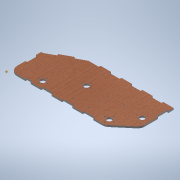
# Autodesk Inventor part: Frame wiel binnen
Saved by Autodesk Inventor 2021 (Build 250183000, 183)
## iProperties
Manager: PJ / DCS
Company: Emmaüs Bovenbouw Aalter
Created: 2020-10-22
Part Number: Frame wiel binnen
Material: S235
Catalog Web Link: http://emmausbovenbouw.op-weg.be/
Vendor: Emmaüsinstituut Bovenbouw Aalter
Document SubType Name: Modeling
Designer: Antho
Engineer: Declercq St.
Manufacturer: Standard
Standards Organization: Custom
Density: 7.86 g/cm^3
Appearance: Steel
Title: Algemene titel
Subject: Specifieke titel
Author: Antho
Keywords: Ruwe Ø xxxxx
Comments: Opmerking
Autodesk Inventor part; units mm, degrees
ref_plane "YZ Plane" through (0, 0, 0) normal (1, 0, 0) x (0, 1, 0)
ref_plane "XZ Plane" through (0, 0, 0) normal (0, 1, 0) x (-1, 0, 0)
ref_plane "XY Plane" through (0, 0, 0) normal (0, 0, 1) x (1, 0, 0)
sketch "Sketch7" plane through (0, 0, 0) normal (0, 0, 1) x (1, 0, 0)
  line L0 (0, 0) -> (0, 51)
  line L1 (340, 102) -> (340, 51)
  line L2 (280, 0) -> (0, 0)
  line L3 (0, 0) -> (0, 30)
  line L4 (280, 0) -> (340, 51)
  line L5 (0, 51) -> (0, 151)
  line L6 (0, 151) -> (340, 151)
  line L7 (340, 102) -> (340, 151)
  line L8 (335, 146) -> (335, 102)
  line L9 (335, 102) -> (335, 53.3122)
  line L10 (335, 53.3122) -> (278.1621, 5)
  line L11 (278.1621, 5) -> (5, 5)
  line L12 (5, 5) -> (5, 51)
  line L13 (5, 51) -> (5, 146)
  line L14 (5, 146) -> (335, 146)
  dimension "d56" = 51
  dimension "d60" = 51
  dimension "d79" = 100
  dimension "d81" = 5
  constraints: 30 end point, 4 perpendicular, 2 vertical, 1 point on line, 6 other
  measures "d56" distance of L0.start L0.end
  measures "d60" distance of L1.start L1.end
  measures "d79" distance of L0.end L5.end
  measures "d81" distance between parallel lines of L6 L14
extrude "Extrusion3" add sketch "Sketch7" along normal blind 5 contours L0 L5 L6 L7 L1 L4 L2 | L8 L9 L10 L11 L12 L13 L14
fillet "Fillet1" radius 25.5 3 edges at (280, 0, 2.5) (340, 51, 2.5) (0, 0, 2.5)
sketch "Sketch9" plane through (0, 0, 5) normal (0, 0, 1) x (1, 0, 0)
  arc A0 (0, 25.5) -> (25.5, 0) centre (25.5, 25.5) ccw projected
  arc A1 (270.6268, 0) -> (287.1418, 6.0705) centre (270.6268, 25.5) ccw projected
  arc A2 (340, 76.5) -> (314.5, 102) centre (314.5, 76.5) ccw projected
  arc A3 (154.2165, 102) -> (146.008, 100.6427) centre (154.2165, 76.5) ccw projected
  point P0 (0, 0)
  constraints: 3 coincident
hole "Hole4" at (154.2165, 76.5, 5) at (314.5, 76.5, 5) at (270.6268, 25.5, 5) direction (0, 0, -1) diameter 15 end through all
sketch "Sketch13" plane through (0, 0, 5) normal (0, 0, 1) x (1, 0, 0)
  circle A0 centre (154.2165, 76.5) radius 7.5 projected
  line L0 (25.5, 25.5) -> (154.2165, 76.5)
  line L1 (154.2165, 76.5) -> (100.2948, 55.1352)
  line L2 (25.5, 25.5) -> (79.4217, 46.8648)
  line L3 (25.5, 25.5) -> (83.5, 25.5)
  line L4 (154.2165, 76.5) -> (154.2165, 18.5)
  circle A1 centre (270.6268, 25.5) radius 7.5 projected
  line L5 (270.6268, 25.5) -> (212.6268, 25.5)
  circle A2 centre (270.6268, 25.5) radius 58
  circle A3 centre (314.5, 76.5) radius 7.5 projected
  circle A4 centre (314.5, 76.5) radius 58
  line L6 (256.7439, 81.814) -> (177.9806, 81.814)
  line L7 (154.2165, 76.5) -> (211.9725, 81.814)
  point P0 (0, 0)
  dimension "d89" = 116
  dimension "d90" = 116
  dimension "d84" = 58
  dimension "d85" = 58
  dimension "d86" = 58
  dimension "d87" = 58
  dimension "d88" = 58
  dimension "d91" = 58
  constraints: 16 end point, 5 coincident, 3 horizontal, 3 point on line, 1 vertical, 6 other
  measures "d84" distance of L0.end L1.end
  measures "d85" distance of L0.start L2.end
  measures "d86" distance of L0.start L3.end
  measures "d87" distance of L0.end L4.end
  measures "d88" distance of L5.start L5.end
  measures "d91" distance of L0.end L7.end
hole "Hole5" at (212.6268, 25.5, 5) at (211.9725, 81.814, 5) at (256.7439, 81.814, 5) direction (0, 0, -1) diameter 4 depth 8
thicken "Thicken1" operation add thickness 5 both sides no extend neighbours yes toward (0, 1, 0) faces at (107.2089, 0, 1.6667) (6.8072, 8.1556, 1.6667) (272.6208, 0.0781, 1.6667) (301.7662, 18.5013, 1.6667) (338.3567, 53.7863, 1.6667) (340, 92.1948, 1.6667) (226.6667, 151, 1.6667) (0, 109.1667, 1.6667)
sketch "Sketch14" plane through (0, 0, 5) normal (0, 0, 1) x (1, 0, 0)
  line L0 (5, 146) -> (5, 25.5) projected
  line L1 (5, 25.5) -> (5, 5)
  line L2 (25.5, 5) -> (270.6268, 5) projected
  line L3 (5, 5) -> (35, 5)
  line L4 (35, 5) -> (65, 5)
  line L5 (65, 5) -> (95, 5)
  line L6 (95, 5) -> (125, 5)
  line L7 (125, 5) -> (155, 5)
  line L8 (155, 5) -> (185, 5)
  line L9 (185, 5) -> (215, 5)
  line L10 (215, 5) -> (245, 5)
  line L11 (245, 5) -> (275, 5)
  line L12 (35, 5) -> (65, 5)
  line L13 (65, 5) -> (65, 10)
  line L14 (65, 10) -> (50, 10)
  line L15 (35, 13) -> (35, 5)
  line L16 (95, 5) -> (125, 5)
  line L17 (125, 5) -> (125, 10)
  line L18 (125, 10) -> (95, 10)
  line L19 (95, 10) -> (95, 5)
  line L20 (155, 5) -> (185, 5)
  line L21 (185, 5) -> (185, 10)
  line L22 (185, 10) -> (155, 10)
  line L23 (155, 10) -> (155, 5)
  line L24 (215, 5) -> (245, 5)
  line L25 (245, 5) -> (245, 10)
  line L26 (245, 10) -> (215, 10)
  line L27 (215, 10) -> (215, 5)
  line L28 (65, 5) -> (50, 5)
  line L29 (50, 5) -> (50, 10)
  line L30 (50, 10) -> (65, 10)
  line L31 (65, 10) -> (65, 5)
  point P0 (0, 0)
  dimension "d102" = 30
  dimension "d103" = 30
  dimension "d104" = 30
  dimension "d105" = 30
  dimension "d106" = 30
  dimension "d107" = 30
  dimension "d109" = 30
  dimension "d110" = 30
  dimension "d111" = 30
  dimension "d113" = 5
  dimension "d114" = 30
  dimension "d115" = 30
  dimension "d118" = 15
  constraints: 60 end point, 12 point on line, 10 parallel, 6 perpendicular, 5 horizontal
  measures "d102" distance of L1.end L3.end
  measures "d103" distance of L3.end L4.end
  measures "d104" distance of L4.end L5.end
  measures "d105" distance of L5.end L6.end
  measures "d106" distance of L6.end L7.end
  measures "d107" distance of L7.end L8.end
  measures "d109" distance of L8.end L9.end
  measures "d110" distance of L9.end L10.end
  measures "d111" distance of L10.end L11.end
  measures "d113" distance of L13.end L12.end
  measures "d114" distance of L18.end L17.end
  measures "d115" distance of L22.end L21.end
  measures "d118" distance of L14.end L30.end
extrude "Extrusion4" cut sketch "Sketch14" against normal blind 10
sketch "Sketch15" plane through (0, 0, 5) normal (0, 0, 1) x (1, 0, 0)
  line L0 (25.5, 5) -> (50, 5) projected
  line L1 (25.5, 5) -> (5, 5)
  arc A0 (5, 25.5) -> (25.5, 5) centre (25.5, 25.5) ccw projected
  line L2 (5, 5) -> (5, 50)
  line L3 (5, 146) -> (5, 25.5) projected
  line L4 (5, 50) -> (5, 80)
  line L5 (5, 80) -> (5, 110)
  line L6 (5, 110) -> (5, 80)
  line L7 (5, 80) -> (5, 110)
  line L8 (5, 110) -> (5, 138)
  line L9 (5, 50) -> (10, 50)
  line L10 (10, 50) -> (10, 80)
  line L11 (10, 80) -> (5, 80)
  line L12 (5, 80) -> (5, 50)
  line L13 (5, 110) -> (10, 110)
  line L14 (10, 110) -> (10, 146)
  line L15 (10, 146) -> (5, 146)
  line L16 (5, 146) -> (5, 110)
  line L17 (5, 110) -> (10, 110)
  line L18 (10, 110) -> (10, 138)
  line L19 (10, 138) -> (5, 138)
  line L20 (5, 138) -> (5, 110)
  point P0 (0, 0)
  point P1 (5, 138)
  dimension "d119" = 45
  dimension "d120" = 30
  dimension "d121" = 30
  dimension "d122" = 30
  dimension "d123" = 30
  dimension "d124" = 28
  dimension "d125" = 5
  dimension "d148" = 28
  constraints: 38 end point, 6 parallel, 6 point on line, 4 horizontal, 3 perpendicular, 2 collinear, 1 tangent
  measures "d119" distance of L1.end L2.end
  measures "d120" distance of L2.end L4.end
  measures "d121" distance of L4.end L5.end
  measures "d122" distance of L5.end L4.end
  measures "d123" distance of L4.end L5.end
  measures "d124" distance of L5.end L8.end
  measures "d125" distance of L11.end L10.end
  measures "d148" distance of L17.end L18.end
extrude "Extrusion5" cut sketch "Sketch15" against normal blind 10 contours L19 L14 L13 L3 | L11 L10 L9 L3
sketch "Sketch16" plane through (0, 0, 5) normal (0, 0, 1) x (1, 0, 0)
  line L0 (335, 146) -> (5, 146) projected
  line L1 (5, 146) -> (35, 146)
  line L2 (35, 146) -> (65, 146)
  line L3 (65, 146) -> (95, 146)
  line L4 (95, 146) -> (125, 146)
  line L5 (125, 146) -> (155, 146)
  line L6 (155, 146) -> (185, 146)
  line L7 (185, 146) -> (215, 146)
  line L8 (215, 146) -> (245, 146)
  line L9 (245, 146) -> (275, 146)
  line L10 (275, 146) -> (305, 146)
  line L11 (305, 146) -> (335, 146)
  line L12 (5, 146) -> (35, 146)
  line L13 (35, 146) -> (35, 141)
  line L14 (35, 141) -> (5, 141)
  line L15 (5, 141) -> (5, 146)
  line L16 (65, 146) -> (95, 146)
  line L17 (95, 146) -> (95, 141)
  line L18 (95, 141) -> (65, 141)
  line L19 (65, 141) -> (65, 146)
  line L20 (125, 146) -> (155, 146)
  line L21 (155, 146) -> (155, 141)
  line L22 (155, 141) -> (125, 141)
  line L23 (125, 141) -> (125, 146)
  line L24 (185, 146) -> (215, 146)
  line L25 (215, 146) -> (215, 141)
  line L26 (215, 141) -> (185, 141)
  line L27 (185, 141) -> (185, 146)
  line L28 (245, 146) -> (275, 146)
  line L29 (275, 146) -> (275, 141)
  line L30 (275, 141) -> (245, 141)
  line L31 (245, 141) -> (245, 146)
  line L32 (335, 62.7922) -> (335, 146) projected
  line L33 (305, 146) -> (335, 146)
  line L34 (335, 146) -> (335, 141)
  line L35 (335, 141) -> (305, 141)
  line L36 (305, 141) -> (305, 146)
  line L37 (35, 146) -> (65, 146)
  line L38 (65, 146) -> (65, 141)
  line L39 (65, 141) -> (35, 141)
  line L40 (35, 141) -> (35, 146)
  line L41 (95, 146) -> (125, 146)
  line L42 (125, 146) -> (125, 141)
  line L43 (125, 141) -> (95, 141)
  line L44 (95, 141) -> (95, 146)
  line L45 (155, 146) -> (185, 146)
  line L46 (185, 146) -> (185, 141)
  line L47 (185, 141) -> (155, 141)
  line L48 (155, 141) -> (155, 146)
  line L49 (215, 146) -> (245, 146)
  line L50 (245, 146) -> (245, 141)
  line L51 (245, 141) -> (215, 141)
  line L52 (215, 141) -> (215, 146)
  line L53 (275, 146) -> (305, 146)
  line L54 (305, 146) -> (305, 141)
  line L55 (305, 141) -> (275, 141)
  line L56 (275, 141) -> (275, 146)
  point P0 (0, 0)
  dimension "d128" = 30
  dimension "d129" = 30
  dimension "d130" = 30
  dimension "d131" = 30
  dimension "d132" = 30
  dimension "d133" = 30
  dimension "d134" = 30
  dimension "d135" = 30
  dimension "d136" = 30
  dimension "d137" = 30
  dimension "d138" = 30
  dimension "d139" = 5
  constraints: 110 end point, 23 equal length, 11 horizontal, 11 perpendicular, 6 point on line, 11 other
  measures "d128" distance of L1.start L1.end
  measures "d129" distance of L1.end L2.end
  measures "d130" distance of L2.end L3.end
  measures "d131" distance of L3.end L4.end
  measures "d132" distance of L4.end L5.end
  measures "d133" distance of L5.end L6.end
  measures "d134" distance of L6.end L7.end
  measures "d135" distance of L7.end L8.end
  measures "d136" distance of L8.end L9.end
  measures "d137" distance of L9.end L10.end
  measures "d138" distance of L10.end L11.end
  measures "d139" distance of L12.end L13.end
extrude "Extrusion6" cut sketch "Sketch16" against normal blind 10 contours L36 L55 L29 L0 | L31 L51 L25 L0 | L27 L47 L21 L0 | L23 L43 L17 L0 | L19 L39 L13 L0
sketch "Sketch17" plane through (0, 0, 5) normal (0, 0, 1) x (1, 0, 0)
  line L0 (335, 146) -> (305, 146) projected
  line L1 (335, 146) -> (335, 131)
  line L2 (335, 62.7922) -> (335, 146) projected
  line L3 (335, 131) -> (335, 101)
  line L4 (335, 101) -> (335, 71)
  line L5 (335, 101) -> (330, 101)
  line L6 (330, 101) -> (330, 131)
  line L7 (330, 131) -> (335, 131)
  line L8 (335, 131) -> (335, 101)
  point P0 (0, 0)
  dimension "d142" = 15
  dimension "d143" = 30
  dimension "d144" = 30
  dimension "d145" = 5
  constraints: 14 end point, 3 point on line, 2 parallel, 1 horizontal, 1 perpendicular
  measures "d142" distance of L0.start L1.end
  measures "d143" distance of L1.end L3.end
  measures "d144" distance of L3.end L4.end
  measures "d145" distance of L6.end L7.end
extrude "Extrusion7" cut sketch "Sketch17" against normal blind 10
sketch "Sketch18" plane through (0, 0, 5) normal (0, 0, 1) x (1, 0, 0)
  circle A0 centre (314.5, 76.5) radius 7.5 projected
  circle A1 centre (314.5, 76.5) radius 16
  line L0 (314.5, 76.5) -> (314.5, 60.5)
  line L1 (314.5, 76.5) -> (298.5, 76.5)
  line L2 (314.5, 76.5) -> (314.5, 92.5)
  point P0 (0, 0)
  dimension "d149" = 32
  constraints: 6 end point, 4 coincident, 3 point on circle, 1 centre point, 1 perpendicular, 1 point on line, 1 vertical
  measures "d149" diameter of A1
hole "Hole6" at (314.5, 92.5, 5) at (298.5, 76.5, 5) at (314.5, 60.5, 5) direction (0, 0, -1) diameter 3 end through all
sketch "Sketch19" plane through (0, 0, 5) normal (0, 0, 1) x (1, 0, 0)
  line L0 (5, 146) -> (5, 138) projected
  line L1 (95, 146) -> (65, 146) projected
  line L2 (5, 146) -> (95, 146)
  line L3 (95, 146) -> (95, 141)
  line L4 (35, 146) -> (5, 146) projected
  line L5 (5, 146) -> (5, 95)
  line L6 (5, 110) -> (5, 80) projected
  line L7 (5, 95) -> (10, 95)
  line L8 (10, 95) -> (37.2636, 109.7544)
  line L9 (95, 141) -> (67.7364, 126.2456)
  line L10 (37.2636, 109.7544) -> (34.8839, 114.1518)
  line L11 (34.8839, 114.1518) -> (65.6654, 130.81)
  line L12 (65.6654, 130.81) -> (68.0452, 126.4127)
  line L13 (10, 95) -> (37.2636, 109.7544)
  line L14 (68.0452, 126.4127) -> (95, 141)
  point P0 (0, 0)
  dimension "d157" = 5
  dimension "d158" = 31
  dimension "d159" = 31
  dimension "d160" = 5
  dimension "d161" = 35
  dimension "d162" = 5
  constraints: 22 end point, 3 perpendicular, 1 collinear, 1 midpoint, 1 point on line
  measures "d157" distance of L5.end L7.end
  measures "d158" distance of L7.end L8.end
  measures "d159" distance of L3.end L9.end
  measures "d160" distance of L8.end L10.end
  measures "d161" distance of L10.end L11.end
  measures "d162" distance of L11.end L12.end
extrude "Extrusion8" cut sketch "Sketch19" against normal blind 5
sketch "Sketch20" plane through (0, 0, 5) normal (0, 0, 1) x (1, 0, 0)
  line L0 (25.5, 25.5) -> (79.4217, 25.5)
  circle A0 centre (79.4217, 25.5) radius 7.5
  point P0 (0, 0)
  dimension "d175" = 15
  constraints: 2 end point, 1 centre point, 1 coincident, 1 horizontal
  measures "d175" diameter of A0
extrude "Extrusion9" cut sketch "Sketch20" against normal blind 10
sketch "Sketch21" plane through (0, 0, 5) normal (0, 0, 1) x (1, 0, 0)
  circle A0 centre (212.6268, 25.5) radius 2 projected
  line L0 (212.6268, 25.5) -> (167.8558, 25.5)
  point P0 (0, 0)
  dimension "d167" = 44.771
  constraints: 2 end point, 1 coincident, 1 horizontal
  measures "d167" distance of L0.start L0.end
hole "Hole7" at (167.8558, 25.5, 5) direction (0, 0, -1) diameter 4 depth 44
sketch "Sketch22" plane through (0, 0, 5) normal (0, 0, 1) x (1, 0, 0)
  circle A0 centre (79.4217, 25.5) radius 7.5 projected
  circle A1 centre (79.4217, 25.5) radius 13
  line L0 (79.4217, 25.5) -> (79.4217, 38.5)
  line L1 (79.4217, 25.5) -> (92.4217, 25.5)
  line L2 (79.4217, 25.5) -> (79.4217, 12.5)
  line L3 (79.4217, 25.5) -> (66.4217, 25.5)
  circle A2 centre (154.2165, 76.5) radius 7.5 projected
  circle A3 centre (154.2165, 76.5) radius 13
  circle A4 centre (270.6268, 25.5) radius 7.5 projected
  circle A5 centre (270.6268, 25.5) radius 13
  line L4 (154.2165, 76.5) -> (154.2165, 89.5)
  line L5 (154.2165, 76.5) -> (167.2165, 76.5)
  line L6 (154.2165, 76.5) -> (154.2165, 63.5)
  line L7 (154.2165, 76.5) -> (141.2165, 76.5)
  line L8 (270.6268, 25.5) -> (270.6268, 38.5)
  line L9 (270.6268, 25.5) -> (283.6268, 25.5)
  line L10 (270.6268, 25.5) -> (270.6268, 12.5)
  line L11 (270.6268, 25.5) -> (257.6268, 25.5)
  point P0 (0, 0)
  dimension "d176" = 26
  dimension "d177" = 26
  dimension "d178" = 26
  constraints: 24 end point, 15 coincident, 12 point on circle, 5 point on line, 4 perpendicular, 3 centre point, 1 vertical
  measures "d176" diameter of A1
  measures "d177" diameter of A3
  measures "d178" diameter of A5
hole "Hole8" at (79.4217, 38.5, 5) at (92.4217, 25.5, 5) at (79.4217, 12.5, 5) at (66.4217, 25.5, 5) at (154.2165, 63.5, 5) at (167.2165, 76.5, 5) at (154.2165, 89.5, 5) at (141.2165, 76.5, 5) at (270.6268, 38.5, 5) at (283.6268, 25.5, 5) at (270.6268, 12.5, 5) at (257.6268, 25.5, 5) direction (0, 0, -1) diameter 4 depth 5
body "Solid2"
